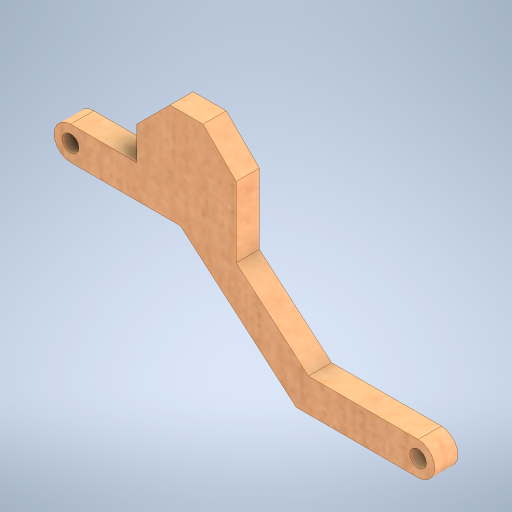
# Autodesk Inventor part: BrazoTV2
Saved by Autodesk Inventor 2023.1 (Build 271208000, 208)
## iProperties
Created: 2022-10-30
Part Number: BrazoTV2
Material: MDF Medium Density Fiberboard
Document SubType Name: Modeling
Designer: Daniel Peña
Density: 0.8 g/cm^3
Appearance: Cherry - Natural Low Gloss
Author: Daniel Peña
Autodesk Inventor part; units mm, degrees
ref_plane "YZ Plane" through (0, 0, 0) normal (1, 0, 0) x (0, 1, 0)
ref_plane "XZ Plane" through (0, 0, 0) normal (0, 1, 0) x (-1, 0, 0)
ref_plane "XY Plane" through (0, 0, 0) normal (0, 0, 1) x (1, 0, 0)
sketch "Sketch1" plane through (0, 0, 0) normal (0, 0, 1) x (1, 0, 0)
  line L0 (-16.7246, 10.0225) -> (18.2754, 10.0225) construction
  line L1 (53.2754, -19.9775) -> (88.2754, -19.9775) construction
  line L2 (18.2754, 10.0225) -> (53.2754, -19.9775) construction
  line L3 (33.2754, 3.7508) -> (55.125, -14.9775)
  line L4 (55.125, -14.9775) -> (88.2754, -14.9775)
  line L5 (-16.7246, 5.0225) -> (16.4258, 5.0225)
  line L6 (16.4258, 5.0225) -> (51.4258, -24.9775)
  line L7 (51.4258, -24.9775) -> (88.2754, -24.9775)
  line L8 (-21.7246, 10.0225) -> (-21.7246, 10.0225)
  line L9 (93.2754, -19.9775) -> (93.2754, -19.9775)
  arc A0 (-21.7246, 10.0225) -> (-16.7246, 5.0225) centre (-16.7246, 10.0225) ccw
  arc A1 (-16.7246, 15.0225) -> (-21.7246, 10.0225) centre (-16.7246, 10.0225) ccw
  arc A2 (88.2754, -24.9775) -> (93.2754, -19.9775) centre (88.2754, -19.9775) ccw
  arc A3 (93.2754, -19.9775) -> (88.2754, -14.9775) centre (88.2754, -19.9775) ccw
  line L10 (33.2754, 3.7508) -> (33.2754, 25.0225)
  line L11 (23.2754, 35.0225) -> (13.2754, 35.0225)
  line L12 (3.2754, 25.0225) -> (3.2754, 15.0225)
  line L13 (18.2754, 10.0225) -> (18.2754, 35.0225) construction
  line L14 (18.2754, 10.0225) -> (43.2754, 10.0225) construction
  line L15 (3.2754, 25.0225) -> (13.2754, 35.0225)
  line L16 (23.2754, 35.0225) -> (33.2754, 25.0225)
  line L17 (-16.7246, 15.0225) -> (3.2754, 15.0225)
  point P0 (0, 0)
  point P1 (25.9584, 10.0225)
  point P2 (93.2754, -19.9775)
  point P3 (33.2754, 35.0225)
  point P4 (3.2754, 35.0225)
  dimension "d0" = 35
  dimension "d4" = 35
  dimension "d5" = 35
  dimension "d6" = 30
  dimension "d8" = 5
  dimension "d10" = 5
  dimension "d11" = 5
  dimension "d12" = 5
  dimension "d22" = 5
  dimension "d23" = 5
  dimension "d24" = 5
  dimension "d25" = 5
  dimension "d26" = 20
  dimension "d29" = 15
  dimension "d30" = 10
  dimension "d31" = 10
  dimension "d32" = 10
  dimension "d33" = 10
  constraints: 36 end point, 8 point on circle, 8 tangent, 5 point on line, 4 centre point, 3 equal radius, 2 horizontal, 2 perpendicular, 2 vertical, 1 midpoint, 1 parallel, 1 other
  measures "d0" distance of L0.start L0.end
  measures "d4" distance of L1.start L1.end
  measures "d5" horizontal distance of L1.start L0.end
  measures "d6" vertical distance of L1.start L0.end
  measures "d8" distance between parallel lines of L0 L5
  measures "d10" distance from line of L0.start L8
  measures "d11" distance from line of L9 L1.end
  measures "d12" radius of A0
  measures "d22" distance between parallel lines of L7 L1
  measures "d23" distance between parallel lines of L4 L1
  measures "d24" distance between parallel lines of L3 L2
  measures "d25" distance between parallel lines of L6 L2
  measures "d26" distance of point (3.275, 35.023) L12.end
  measures "d29" distance between parallel lines of L12 L13
  measures "d30" distance of L12.start point (3.275, 35.023)
  measures "d31" distance of L11.end point (3.275, 35.023)
  measures "d32" distance of L11.start point (33.275, 35.023)
  measures "d33" distance of L10.end point (33.275, 35.023)
extrude "Extrusion1" add sketch "Sketch1" along normal blind 7
sketch "Sketch2" plane through (0, 0, 7) normal (0, 0, 1) x (1, 0, 0)
  arc A0 (-16.7246, 15.0225) -> (-16.7246, 5.0225) centre (-16.7246, 10.0225) ccw projected
  arc A1 (88.2754, -24.9775) -> (88.2754, -14.9775) centre (88.2754, -19.9775) ccw projected
  point P0 (0, 0)
  constraints: 2 coincident
hole "Hole1" at (-16.7246, 10.0225, 7) at (88.2754, -19.9775, 7) direction (0, 0, -1) diameter 5 end through all
equation "\"d31\" = d30"
equation "\"d32\" = d30"
equation "\"d33\" = d32"
body "Solid1"
